Autodesk Inventor part; units mm, degrees
(part 3 of 4)
sketch "Sketch4" plane through (0, 2, 0) normal (0, 1, 0) x (1, 0, 0)
  line L0 (-144.19, 379.14) -> (-144.19, 0) projected
  line L1 (0, 379.14) -> (-144.19, 379.14) projected
  line L2 (-131.665, 24.5025) -> (-131.665, 37.5025)
  line L3 (-117.665, 24.5025) -> (-117.665, 37.5025)
  line L4 (-131.165, 24.0025) -> (-118.165, 24.0025)
  line L5 (-131.165, 38.0025) -> (-118.165, 38.0025)
  arc A0 (-131.665, 24.5025) -> (-131.165, 24.0025) centre (-131.165, 24.5025) ccw
  arc A1 (-131.165, 38.0025) -> (-131.665, 37.5025) centre (-131.165, 37.5025) ccw
  arc A2 (-118.165, 24.0025) -> (-117.665, 24.5025) centre (-118.165, 24.5025) ccw
  arc A3 (-117.665, 37.5025) -> (-118.165, 38.0025) centre (-118.165, 37.5025) ccw
  line L6 (-131.665, 62.6025) -> (-131.665, 75.6025)
  line L7 (-117.665, 62.6025) -> (-117.665, 75.6025)
  line L8 (-131.165, 62.1025) -> (-118.165, 62.1025)
  line L9 (-131.165, 76.1025) -> (-118.165, 76.1025)
  arc A4 (-131.665, 62.6025) -> (-131.165, 62.1025) centre (-131.165, 62.6025) ccw
  arc A5 (-131.165, 76.1025) -> (-131.665, 75.6025) centre (-131.165, 75.6025) ccw
  arc A6 (-118.165, 62.1025) -> (-117.665, 62.6025) centre (-118.165, 62.6025) ccw
  arc A7 (-117.665, 75.6025) -> (-118.165, 76.1025) centre (-118.165, 75.6025) ccw
  line L10 (-131.665, 81.6525) -> (-131.665, 94.6525)
  line L11 (-117.665, 81.6525) -> (-117.665, 94.6525)
  line L12 (-131.165, 81.1525) -> (-118.165, 81.1525)
  line L13 (-131.165, 95.1525) -> (-118.165, 95.1525)
  arc A8 (-131.665, 81.6525) -> (-131.165, 81.1525) centre (-131.165, 81.6525) ccw
  arc A9 (-131.165, 95.1525) -> (-131.665, 94.6525) centre (-131.165, 94.6525) ccw
  arc A10 (-118.165, 81.1525) -> (-117.665, 81.6525) centre (-118.165, 81.6525) ccw
  arc A11 (-117.665, 94.6525) -> (-118.165, 95.1525) centre (-118.165, 94.6525) ccw
  line L14 (-131.665, 100.7025) -> (-131.665, 113.7025)
  line L15 (-117.665, 100.7025) -> (-117.665, 113.7025)
  line L16 (-131.165, 100.2025) -> (-118.165, 100.2025)
  line L17 (-131.165, 114.2025) -> (-118.165, 114.2025)
  arc A12 (-131.665, 100.7025) -> (-131.165, 100.2025) centre (-131.165, 100.7025) ccw
  arc A13 (-131.165, 114.2025) -> (-131.665, 113.7025) centre (-131.165, 113.7025) ccw
  arc A14 (-118.165, 100.2025) -> (-117.665, 100.7025) centre (-118.165, 100.7025) ccw
  arc A15 (-117.665, 113.7025) -> (-118.165, 114.2025) centre (-118.165, 113.7025) ccw
  line L18 (-131.665, 119.7525) -> (-131.665, 132.7525)
  line L19 (-117.665, 119.7525) -> (-117.665, 132.7525)
  line L20 (-131.165, 119.2525) -> (-118.165, 119.2525)
  line L21 (-131.165, 133.2525) -> (-118.165, 133.2525)
  arc A16 (-131.665, 119.7525) -> (-131.165, 119.2525) centre (-131.165, 119.7525) ccw
  arc A17 (-131.165, 133.2525) -> (-131.665, 132.7525) centre (-131.165, 132.7525) ccw
  arc A18 (-118.165, 119.2525) -> (-117.665, 119.7525) centre (-118.165, 119.7525) ccw
  arc A19 (-117.665, 132.7525) -> (-118.165, 133.2525) centre (-118.165, 132.7525) ccw
  line L22 (-131.665, 148.3275) -> (-131.665, 161.3275)
  line L23 (-117.665, 148.3275) -> (-117.665, 161.3275)
  line L24 (-131.165, 147.8275) -> (-118.165, 147.8275)
  line L25 (-131.165, 161.8275) -> (-118.165, 161.8275)
  arc A20 (-131.665, 148.3275) -> (-131.165, 147.8275) centre (-131.165, 148.3275) ccw
  arc A21 (-131.165, 161.8275) -> (-131.665, 161.3275) centre (-131.165, 161.3275) ccw
  arc A22 (-118.165, 147.8275) -> (-117.665, 148.3275) centre (-118.165, 148.3275) ccw
  arc A23 (-117.665, 161.3275) -> (-118.165, 161.8275) centre (-118.165, 161.3275) ccw
  line L26 (-131.665, 167.3775) -> (-131.665, 180.3775)
  line L27 (-117.665, 167.3775) -> (-117.665, 180.3775)
  line L28 (-131.165, 166.8775) -> (-118.165, 166.8775)
  line L29 (-131.165, 180.8775) -> (-118.165, 180.8775)
  arc A24 (-131.665, 167.3775) -> (-131.165, 166.8775) centre (-131.165, 167.3775) ccw
  arc A25 (-131.165, 180.8775) -> (-131.665, 180.3775) centre (-131.165, 180.3775) ccw
  arc A26 (-118.165, 166.8775) -> (-117.665, 167.3775) centre (-118.165, 167.3775) ccw
  arc A27 (-117.665, 180.3775) -> (-118.165, 180.8775) centre (-118.165, 180.3775) ccw
  line L30 (-131.665, 186.4275) -> (-131.665, 199.4275)
  line L31 (-117.665, 186.4275) -> (-117.665, 199.4275)
  line L32 (-131.165, 185.9275) -> (-118.165, 185.9275)
  line L33 (-131.165, 199.9275) -> (-118.165, 199.9275)
  arc A28 (-131.665, 186.4275) -> (-131.165, 185.9275) centre (-131.165, 186.4275) ccw
  arc A29 (-131.165, 199.9275) -> (-131.665, 199.4275) centre (-131.165, 199.4275) ccw
  arc A30 (-118.165, 185.9275) -> (-117.665, 186.4275) centre (-118.165, 186.4275) ccw
  arc A31 (-117.665, 199.4275) -> (-118.165, 199.9275) centre (-118.165, 199.4275) ccw
  line L34 (-131.665, 205.4775) -> (-131.665, 218.4775)
  line L35 (-117.665, 205.4775) -> (-117.665, 218.4775)
  line L36 (-131.165, 204.9775) -> (-118.165, 204.9775)
  line L37 (-131.165, 218.9775) -> (-118.165, 218.9775)
  arc A32 (-131.665, 205.4775) -> (-131.165, 204.9775) centre (-131.165, 205.4775) ccw
  arc A33 (-131.165, 218.9775) -> (-131.665, 218.4775) centre (-131.165, 218.4775) ccw
  arc A34 (-118.165, 204.9775) -> (-117.665, 205.4775) centre (-118.165, 205.4775) ccw
  arc A35 (-117.665, 218.4775) -> (-118.165, 218.9775) centre (-118.165, 218.4775) ccw
  line L38 (-131.665, 234.0525) -> (-131.665, 247.0525)
  line L39 (-117.665, 234.0525) -> (-117.665, 247.0525)
  line L40 (-131.165, 233.5525) -> (-118.165, 233.5525)
  line L41 (-131.165, 247.5525) -> (-118.165, 247.5525)
  arc A36 (-131.665, 234.0525) -> (-131.165, 233.5525) centre (-131.165, 234.0525) ccw
  arc A37 (-131.165, 247.5525) -> (-131.665, 247.0525) centre (-131.165, 247.0525) ccw
  arc A38 (-118.165, 233.5525) -> (-117.665, 234.0525) centre (-118.165, 234.0525) ccw
  arc A39 (-117.665, 247.0525) -> (-118.165, 247.5525) centre (-118.165, 247.0525) ccw
  line L42 (-131.665, 253.1025) -> (-131.665, 266.1025)
  line L43 (-117.665, 253.1025) -> (-117.665, 266.1025)
  line L44 (-131.165, 252.6025) -> (-118.165, 252.6025)
  line L45 (-131.165, 266.6025) -> (-118.165, 266.6025)
  arc A40 (-131.665, 253.1025) -> (-131.165, 252.6025) centre (-131.165, 253.1025) ccw
  arc A41 (-131.165, 266.6025) -> (-131.665, 266.1025) centre (-131.165, 266.1025) ccw
  arc A42 (-118.165, 252.6025) -> (-117.665, 253.1025) centre (-118.165, 253.1025) ccw
  arc A43 (-117.665, 266.1025) -> (-118.165, 266.6025) centre (-118.165, 266.1025) ccw
  line L46 (-131.665, 272.1525) -> (-131.665, 285.1525)
  line L47 (-117.665, 272.1525) -> (-117.665, 285.1525)
  line L48 (-131.165, 271.6525) -> (-118.165, 271.6525)
  line L49 (-131.165, 285.6525) -> (-118.165, 285.6525)
  arc A44 (-131.665, 272.1525) -> (-131.165, 271.6525) centre (-131.165, 272.1525) ccw
  arc A45 (-131.165, 285.6525) -> (-131.665, 285.1525) centre (-131.165, 285.1525) ccw
  arc A46 (-118.165, 271.6525) -> (-117.665, 272.1525) centre (-118.165, 272.1525) ccw
  arc A47 (-117.665, 285.1525) -> (-118.165, 285.6525) centre (-118.165, 285.1525) ccw
  line L50 (-131.665, 291.2025) -> (-131.665, 304.2025)
  line L51 (-117.665, 291.2025) -> (-117.665, 304.2025)
  line L52 (-131.165, 290.7025) -> (-118.165, 290.7025)
  line L53 (-131.165, 304.7025) -> (-118.165, 304.7025)
  arc A48 (-131.665, 291.2025) -> (-131.165, 290.7025) centre (-131.165, 291.2025) ccw
  arc A49 (-131.165, 304.7025) -> (-131.665, 304.2025) centre (-131.165, 304.2025) ccw
  arc A50 (-118.165, 290.7025) -> (-117.665, 291.2025) centre (-118.165, 291.2025) ccw
  arc A51 (-117.665, 304.2025) -> (-118.165, 304.7025) centre (-118.165, 304.2025) ccw
  line L54 (-107.8525, 24.5025) -> (-107.8525, 37.5025)
  line L55 (-93.8525, 24.5025) -> (-93.8525, 37.5025)
  line L56 (-107.3525, 24.0025) -> (-94.3525, 24.0025)
  line L57 (-107.3525, 38.0025) -> (-94.3525, 38.0025)
  arc A52 (-107.8525, 24.5025) -> (-107.3525, 24.0025) centre (-107.3525, 24.5025) ccw
  arc A53 (-107.3525, 38.0025) -> (-107.8525, 37.5025) centre (-107.3525, 37.5025) ccw
  arc A54 (-94.3525, 24.0025) -> (-93.8525, 24.5025) centre (-94.3525, 24.5025) ccw
  arc A55 (-93.8525, 37.5025) -> (-94.3525, 38.0025) centre (-94.3525, 37.5025) ccw
  line L58 (-107.8525, 43.5525) -> (-107.8525, 56.5525)
  line L59 (-93.8525, 43.5525) -> (-93.8525, 56.5525)
  line L60 (-107.3525, 43.0525) -> (-94.3525, 43.0525)
  line L61 (-107.3525, 57.0525) -> (-94.3525, 57.0525)
  arc A56 (-107.8525, 43.5525) -> (-107.3525, 43.0525) centre (-107.3525, 43.5525) ccw
  arc A57 (-107.3525, 57.0525) -> (-107.8525, 56.5525) centre (-107.3525, 56.5525) ccw
  arc A58 (-94.3525, 43.0525) -> (-93.8525, 43.5525) centre (-94.3525, 43.5525) ccw
  arc A59 (-93.8525, 56.5525) -> (-94.3525, 57.0525) centre (-94.3525, 56.5525) ccw
  line L62 (-107.8525, 62.6025) -> (-107.8525, 75.6025)
  line L63 (-93.8525, 62.6025) -> (-93.8525, 75.6025)
  line L64 (-107.3525, 62.1025) -> (-94.3525, 62.1025)
  line L65 (-107.3525, 76.1025) -> (-94.3525, 76.1025)
  arc A60 (-107.8525, 62.6025) -> (-107.3525, 62.1025) centre (-107.3525, 62.6025) ccw
  arc A61 (-107.3525, 76.1025) -> (-107.8525, 75.6025) centre (-107.3525, 75.6025) ccw
  arc A62 (-94.3525, 62.1025) -> (-93.8525, 62.6025) centre (-94.3525, 62.6025) ccw
  arc A63 (-93.8525, 75.6025) -> (-94.3525, 76.1025) centre (-94.3525, 75.6025) ccw
  line L66 (-107.8525, 81.6525) -> (-107.8525, 94.6525)
  line L67 (-93.8525, 81.6525) -> (-93.8525, 94.6525)
  line L68 (-107.3525, 81.1525) -> (-94.3525, 81.1525)
  line L69 (-107.3525, 95.1525) -> (-94.3525, 95.1525)
  arc A64 (-107.8525, 81.6525) -> (-107.3525, 81.1525) centre (-107.3525, 81.6525) ccw
  arc A65 (-107.3525, 95.1525) -> (-107.8525, 94.6525) centre (-107.3525, 94.6525) ccw
  arc A66 (-94.3525, 81.1525) -> (-93.8525, 81.6525) centre (-94.3525, 81.6525) ccw
  arc A67 (-93.8525, 94.6525) -> (-94.3525, 95.1525) centre (-94.3525, 94.6525) ccw
  line L70 (-107.8525, 100.7025) -> (-107.8525, 113.7025)
  line L71 (-93.8525, 100.7025) -> (-93.8525, 113.7025)
  line L72 (-107.3525, 100.2025) -> (-94.3525, 100.2025)
  line L73 (-107.3525, 114.2025) -> (-94.3525, 114.2025)
  arc A68 (-107.8525, 100.7025) -> (-107.3525, 100.2025) centre (-107.3525, 100.7025) ccw
  arc A69 (-107.3525, 114.2025) -> (-107.8525, 113.7025) centre (-107.3525, 113.7025) ccw
  arc A70 (-94.3525, 100.2025) -> (-93.8525, 100.7025) centre (-94.3525, 100.7025) ccw
  arc A71 (-93.8525, 113.7025) -> (-94.3525, 114.2025) centre (-94.3525, 113.7025) ccw
  line L74 (-107.8525, 119.7525) -> (-107.8525, 132.7525)
  line L75 (-93.8525, 119.7525) -> (-93.8525, 132.7525)
  line L76 (-107.3525, 119.2525) -> (-94.3525, 119.2525)
  line L77 (-107.3525, 133.2525) -> (-94.3525, 133.2525)
  arc A72 (-107.8525, 119.7525) -> (-107.3525, 119.2525) centre (-107.3525, 119.7525) ccw
  arc A73 (-107.3525, 133.2525) -> (-107.8525, 132.7525) centre (-107.3525, 132.7525) ccw
  arc A74 (-94.3525, 119.2525) -> (-93.8525, 119.7525) centre (-94.3525, 119.7525) ccw
  arc A75 (-93.8525, 132.7525) -> (-94.3525, 133.2525) centre (-94.3525, 132.7525) ccw
  line L78 (-107.8525, 138.8025) -> (-107.8525, 151.8025)
  line L79 (-93.8525, 138.8025) -> (-93.8525, 151.8025)
  line L80 (-107.3525, 138.3025) -> (-94.3525, 138.3025)
  line L81 (-107.3525, 152.3025) -> (-94.3525, 152.3025)
  arc A76 (-107.8525, 138.8025) -> (-107.3525, 138.3025) centre (-107.3525, 138.8025) ccw
  arc A77 (-107.3525, 152.3025) -> (-107.8525, 151.8025) centre (-107.3525, 151.8025) ccw
  arc A78 (-94.3525, 138.3025) -> (-93.8525, 138.8025) centre (-94.3525, 138.8025) ccw
  arc A79 (-93.8525, 151.8025) -> (-94.3525, 152.3025) centre (-94.3525, 151.8025) ccw
  line L82 (-107.8525, 157.8525) -> (-107.8525, 170.8525)
  line L83 (-93.8525, 157.8525) -> (-93.8525, 170.8525)
  line L84 (-107.3525, 157.3525) -> (-94.3525, 157.3525)
  line L85 (-107.3525, 171.3525) -> (-94.3525, 171.3525)
  arc A80 (-107.8525, 157.8525) -> (-107.3525, 157.3525) centre (-107.3525, 157.8525) ccw
  arc A81 (-107.3525, 171.3525) -> (-107.8525, 170.8525) centre (-107.3525, 170.8525) ccw
  arc A82 (-94.3525, 157.3525) -> (-93.8525, 157.8525) centre (-94.3525, 157.8525) ccw
  arc A83 (-93.8525, 170.8525) -> (-94.3525, 171.3525) centre (-94.3525, 170.8525) ccw
  line L86 (-107.8525, 176.9025) -> (-107.8525, 189.9025)
  line L87 (-93.8525, 176.9025) -> (-93.8525, 189.9025)
  line L88 (-107.3525, 176.4025) -> (-94.3525, 176.4025)
  line L89 (-107.3525, 190.4025) -> (-94.3525, 190.4025)
  arc A84 (-107.8525, 176.9025) -> (-107.3525, 176.4025) centre (-107.3525, 176.9025) ccw
  arc A85 (-107.3525, 190.4025) -> (-107.8525, 189.9025) centre (-107.3525, 189.9025) ccw
  arc A86 (-94.3525, 176.4025) -> (-93.8525, 176.9025) centre (-94.3525, 176.9025) ccw
  arc A87 (-93.8525, 189.9025) -> (-94.3525, 190.4025) centre (-94.3525, 189.9025) ccw
  line L90 (-107.8525, 195.9525) -> (-107.8525, 208.9525)
  line L91 (-93.8525, 195.9525) -> (-93.8525, 208.9525)
  line L92 (-107.3525, 195.4525) -> (-94.3525, 195.4525)
  line L93 (-107.3525, 209.4525) -> (-94.3525, 209.4525)
  arc A88 (-107.8525, 195.9525) -> (-107.3525, 195.4525) centre (-107.3525, 195.9525) ccw
  arc A89 (-107.3525, 209.4525) -> (-107.8525, 208.9525) centre (-107.3525, 208.9525) ccw
  arc A90 (-94.3525, 195.4525) -> (-93.8525, 195.9525) centre (-94.3525, 195.9525) ccw
  arc A91 (-93.8525, 208.9525) -> (-94.3525, 209.4525) centre (-94.3525, 208.9525) ccw
  line L94 (-107.8525, 215.0025) -> (-107.8525, 228.0025)
  line L95 (-93.8525, 215.0025) -> (-93.8525, 228.0025)
  line L96 (-107.3525, 214.5025) -> (-94.3525, 214.5025)
  line L97 (-107.3525, 228.5025) -> (-94.3525, 228.5025)
  arc A92 (-107.8525, 215.0025) -> (-107.3525, 214.5025) centre (-107.3525, 215.0025) ccw
  arc A93 (-107.3525, 228.5025) -> (-107.8525, 228.0025) centre (-107.3525, 228.0025) ccw
  arc A94 (-94.3525, 214.5025) -> (-93.8525, 215.0025) centre (-94.3525, 215.0025) ccw
  arc A95 (-93.8525, 228.0025) -> (-94.3525, 228.5025) centre (-94.3525, 228.0025) ccw
  line L98 (-107.8525, 234.0525) -> (-107.8525, 247.0525)
  line L99 (-93.8525, 234.0525) -> (-93.8525, 247.0525)
  line L100 (-107.3525, 233.5525) -> (-94.3525, 233.5525)
  line L101 (-107.3525, 247.5525) -> (-94.3525, 247.5525)
  arc A96 (-107.8525, 234.0525) -> (-107.3525, 233.5525) centre (-107.3525, 234.0525) ccw
  arc A97 (-107.3525, 247.5525) -> (-107.8525, 247.0525) centre (-107.3525, 247.0525) ccw
  arc A98 (-94.3525, 233.5525) -> (-93.8525, 234.0525) centre (-94.3525, 234.0525) ccw
  arc A99 (-93.8525, 247.0525) -> (-94.3525, 247.5525) centre (-94.3525, 247.0525) ccw
  line L102 (-107.8525, 253.1025) -> (-107.8525, 266.1025)
  line L103 (-93.8525, 253.1025) -> (-93.8525, 266.1025)
  line L104 (-107.3525, 252.6025) -> (-94.3525, 252.6025)
  line L105 (-107.3525, 266.6025) -> (-94.3525, 266.6025)
  arc A100 (-107.8525, 253.1025) -> (-107.3525, 252.6025) centre (-107.3525, 253.1025) ccw
  arc A101 (-107.3525, 266.6025) -> (-107.8525, 266.1025) centre (-107.3525, 266.1025) ccw
  arc A102 (-94.3525, 252.6025) -> (-93.8525, 253.1025) centre (-94.3525, 253.1025) ccw
  arc A103 (-93.8525, 266.1025) -> (-94.3525, 266.6025) centre (-94.3525, 266.1025) ccw
  line L106 (-107.8525, 281.6775) -> (-107.8525, 294.6775)
  line L107 (-93.8525, 281.6775) -> (-93.8525, 294.6775)
  line L108 (-107.3525, 281.1775) -> (-94.3525, 281.1775)
  line L109 (-107.3525, 295.1775) -> (-94.3525, 295.1775)
  arc A104 (-107.8525, 281.6775) -> (-107.3525, 281.1775) centre (-107.3525, 281.6775) ccw
  arc A105 (-107.3525, 295.1775) -> (-107.8525, 294.6775) centre (-107.3525, 294.6775) ccw
  arc A106 (-94.3525, 281.1775) -> (-93.8525, 281.6775) centre (-94.3525, 281.6775) ccw
  arc A107 (-93.8525, 294.6775) -> (-94.3525, 295.1775) centre (-94.3525, 294.6775) ccw
  line L110 (-106.8525, 273.2395) -> (-106.8525, 279.2395)
  line L111 (-91.8525, 273.2395) -> (-91.8525, 279.2395)
  line L112 (-106.3525, 272.7395) -> (-92.3525, 272.7395)
  line L113 (-106.3525, 279.7395) -> (-92.3525, 279.7395)
  arc A108 (-106.8525, 273.2395) -> (-106.3525, 272.7395) centre (-106.3525, 273.2395) ccw
  arc A109 (-106.3525, 279.7395) -> (-106.8525, 279.2395) centre (-106.3525, 279.2395) ccw
  arc A110 (-92.3525, 272.7395) -> (-91.8525, 273.2395) centre (-92.3525, 273.2395) ccw
  arc A111 (-91.8525, 279.2395) -> (-92.3525, 279.7395) centre (-92.3525, 279.2395) ccw
  line L114 (-106.8525, 297.1155) -> (-106.8525, 303.1155)
  line L115 (-91.8525, 297.1155) -> (-91.8525, 303.1155)
  line L116 (-106.3525, 296.6155) -> (-92.3525, 296.6155)
  line L117 (-106.3525, 303.6155) -> (-92.3525, 303.6155)
  arc A112 (-106.8525, 297.1155) -> (-106.3525, 296.6155) centre (-106.3525, 297.1155) ccw
  arc A113 (-106.3525, 303.6155) -> (-106.8525, 303.1155) centre (-106.3525, 303.1155) ccw
  arc A114 (-92.3525, 296.6155) -> (-91.8525, 297.1155) centre (-92.3525, 297.1155) ccw
  arc A115 (-91.8525, 303.1155) -> (-92.3525, 303.6155) centre (-92.3525, 303.1155) ccw
  line L118 (-107.8525, 315.015) -> (-107.8525, 328.015)
  line L119 (-93.8525, 315.015) -> (-93.8525, 328.015)
  line L120 (-107.3525, 314.515) -> (-94.3525, 314.515)
  line L121 (-107.3525, 328.515) -> (-94.3525, 328.515)
  arc A116 (-107.8525, 315.015) -> (-107.3525, 314.515) centre (-107.3525, 315.015) ccw
  arc A117 (-107.3525, 328.515) -> (-107.8525, 328.015) centre (-107.3525, 328.015) ccw
  arc A118 (-94.3525, 314.515) -> (-93.8525, 315.015) centre (-94.3525, 315.015) ccw
  arc A119 (-93.8525, 328.015) -> (-94.3525, 328.515) centre (-94.3525, 328.015) ccw
  line L122 (-107.8525, 334.065) -> (-107.8525, 347.065)
  line L123 (-93.8525, 334.065) -> (-93.8525, 347.065)
  line L124 (-107.3525, 333.565) -> (-94.3525, 333.565)
  line L125 (-107.3525, 347.565) -> (-94.3525, 347.565)
  arc A120 (-107.8525, 334.065) -> (-107.3525, 333.565) centre (-107.3525, 334.065) ccw
  arc A121 (-107.3525, 347.565) -> (-107.8525, 347.065) centre (-107.3525, 347.065) ccw
  arc A122 (-94.3525, 333.565) -> (-93.8525, 334.065) centre (-94.3525, 334.065) ccw
  arc A123 (-93.8525, 347.065) -> (-94.3525, 347.565) centre (-94.3525, 347.065) ccw
  line L126 (-107.8525, 353.115) -> (-107.8525, 366.115)
  line L127 (-93.8525, 353.115) -> (-93.8525, 366.115)
  line L128 (-107.3525, 352.615) -> (-94.3525, 352.615)
  line L129 (-107.3525, 366.615) -> (-94.3525, 366.615)
  arc A124 (-107.8525, 353.115) -> (-107.3525, 352.615) centre (-107.3525, 353.115) ccw
  arc A125 (-107.3525, 366.615) -> (-107.8525, 366.115) centre (-107.3525, 366.115) ccw
  arc A126 (-94.3525, 352.615) -> (-93.8525, 353.115) centre (-94.3525, 353.115) ccw
  arc A127 (-93.8525, 366.115) -> (-94.3525, 366.615) centre (-94.3525, 366.115) ccw
  line L130 (-88.8025, 29.265) -> (-88.8025, 42.265)
  line L131 (-74.8025, 29.265) -> (-74.8025, 42.265)
  line L132 (-88.3025, 28.765) -> (-75.3025, 28.765)
  line L133 (-88.3025, 42.765) -> (-75.3025, 42.765)
  arc A128 (-88.8025, 29.265) -> (-88.3025, 28.765) centre (-88.3025, 29.265) ccw
  arc A129 (-88.3025, 42.765) -> (-88.8025, 42.265) centre (-88.3025, 42.265) ccw
  arc A130 (-75.3025, 28.765) -> (-74.8025, 29.265) centre (-75.3025, 29.265) ccw
  arc A131 (-74.8025, 42.265) -> (-75.3025, 42.765) centre (-75.3025, 42.265) ccw
  line L134 (-88.8025, 53.0775) -> (-88.8025, 66.0775)
  line L135 (-74.8025, 53.0775) -> (-74.8025, 66.0775)
  line L136 (-88.3025, 52.5775) -> (-75.3025, 52.5775)
  line L137 (-88.3025, 66.5775) -> (-75.3025, 66.5775)
  arc A132 (-88.8025, 53.0775) -> (-88.3025, 52.5775) centre (-88.3025, 53.0775) ccw
  arc A133 (-88.3025, 66.5775) -> (-88.8025, 66.0775) centre (-88.3025, 66.0775) ccw
  arc A134 (-75.3025, 52.5775) -> (-74.8025, 53.0775) centre (-75.3025, 53.0775) ccw
  arc A135 (-74.8025, 66.0775) -> (-75.3025, 66.5775) centre (-75.3025, 66.0775) ccw
  line L138 (-88.8025, 72.1275) -> (-88.8025, 85.1275)
  line L139 (-74.8025, 72.1275) -> (-74.8025, 85.1275)
  line L140 (-88.3025, 71.6275) -> (-75.3025, 71.6275)
  line L141 (-88.3025, 85.6275) -> (-75.3025, 85.6275)
  arc A136 (-88.8025, 72.1275) -> (-88.3025, 71.6275) centre (-88.3025, 72.1275) ccw
  arc A137 (-88.3025, 85.6275) -> (-88.8025, 85.1275) centre (-88.3025, 85.1275) ccw
  arc A138 (-75.3025, 71.6275) -> (-74.8025, 72.1275) centre (-75.3025, 72.1275) ccw
  arc A139 (-74.8025, 85.1275) -> (-75.3025, 85.6275) centre (-75.3025, 85.1275) ccw
  line L142 (-88.8025, 91.1775) -> (-88.8025, 104.1775)
  line L143 (-74.8025, 91.1775) -> (-74.8025, 104.1775)
  line L144 (-88.3025, 90.6775) -> (-75.3025, 90.6775)
  line L145 (-88.3025, 104.6775) -> (-75.3025, 104.6775)
  arc A140 (-88.8025, 91.1775) -> (-88.3025, 90.6775) centre (-88.3025, 91.1775) ccw
  arc A141 (-88.3025, 104.6775) -> (-88.8025, 104.1775) centre (-88.3025, 104.1775) ccw
  arc A142 (-75.3025, 90.6775) -> (-74.8025, 91.1775) centre (-75.3025, 91.1775) ccw
  arc A143 (-74.8025, 104.1775) -> (-75.3025, 104.6775) centre (-75.3025, 104.1775) ccw
  line L146 (-88.8025, 110.2275) -> (-88.8025, 123.2275)
  line L147 (-74.8025, 110.2275) -> (-74.8025, 123.2275)
  line L148 (-88.3025, 109.7275) -> (-75.3025, 109.7275)
  line L149 (-88.3025, 123.7275) -> (-75.3025, 123.7275)
  arc A144 (-88.8025, 110.2275) -> (-88.3025, 109.7275) centre (-88.3025, 110.2275) ccw
  arc A145 (-88.3025, 123.7275) -> (-88.8025, 123.2275) centre (-88.3025, 123.2275) ccw
  arc A146 (-75.3025, 109.7275) -> (-74.8025, 110.2275) centre (-75.3025, 110.2275) ccw
  arc A147 (-74.8025, 123.2275) -> (-75.3025, 123.7275) centre (-75.3025, 123.2275) ccw
  line L150 (-88.8025, 129.2775) -> (-88.8025, 142.2775)
  line L151 (-74.8025, 129.2775) -> (-74.8025, 142.2775)
  line L152 (-88.3025, 128.7775) -> (-75.3025, 128.7775)
  line L153 (-88.3025, 142.7775) -> (-75.3025, 142.7775)
  arc A148 (-88.8025, 129.2775) -> (-88.3025, 128.7775) centre (-88.3025, 129.2775) ccw
  arc A149 (-88.3025, 142.7775) -> (-88.8025, 142.2775) centre (-88.3025, 142.2775) ccw
  arc A150 (-75.3025, 128.7775) -> (-74.8025, 129.2775) centre (-75.3025, 129.2775) ccw
  arc A151 (-74.8025, 142.2775) -> (-75.3025, 142.7775) centre (-75.3025, 142.2775) ccw
  line L154 (-88.8025, 148.3275) -> (-88.8025, 161.3275)
  line L155 (-74.8025, 148.3275) -> (-74.8025, 161.3275)
  line L156 (-88.3025, 147.8275) -> (-75.3025, 147.8275)
  line L157 (-88.3025, 161.8275) -> (-75.3025, 161.8275)
  arc A152 (-88.8025, 148.3275) -> (-88.3025, 147.8275) centre (-88.3025, 148.3275) ccw
  arc A153 (-88.3025, 161.8275) -> (-88.8025, 161.3275) centre (-88.3025, 161.3275) ccw
  arc A154 (-75.3025, 147.8275) -> (-74.8025, 148.3275) centre (-75.3025, 148.3275) ccw
  arc A155 (-74.8025, 161.3275) -> (-75.3025, 161.8275) centre (-75.3025, 161.3275) ccw
  line L158 (-88.8025, 167.3775) -> (-88.8025, 180.3775)
  line L159 (-74.8025, 167.3775) -> (-74.8025, 180.3775)
  line L160 (-88.3025, 166.8775) -> (-75.3025, 166.8775)
  line L161 (-88.3025, 180.8775) -> (-75.3025, 180.8775)
  arc A156 (-88.8025, 167.3775) -> (-88.3025, 166.8775) centre (-88.3025, 167.3775) ccw
  arc A157 (-88.3025, 180.8775) -> (-88.8025, 180.3775) centre (-88.3025, 180.3775) ccw
  arc A158 (-75.3025, 166.8775) -> (-74.8025, 167.3775) centre (-75.3025, 167.3775) ccw
  arc A159 (-74.8025, 180.3775) -> (-75.3025, 180.8775) centre (-75.3025, 180.3775) ccw
  line L162 (-88.8025, 186.4275) -> (-88.8025, 199.4275)
  line L163 (-74.8025, 186.4275) -> (-74.8025, 199.4275)
  line L164 (-88.3025, 185.9275) -> (-75.3025, 185.9275)
  line L165 (-88.3025, 199.9275) -> (-75.3025, 199.9275)
  arc A160 (-88.8025, 186.4275) -> (-88.3025, 185.9275) centre (-88.3025, 186.4275) ccw
  arc A161 (-88.3025, 199.9275) -> (-88.8025, 199.4275) centre (-88.3025, 199.4275) ccw
  arc A162 (-75.3025, 185.9275) -> (-74.8025, 186.4275) centre (-75.3025, 186.4275) ccw
  arc A163 (-74.8025, 199.4275) -> (-75.3025, 199.9275) centre (-75.3025, 199.4275) ccw
  line L166 (-88.8025, 205.4775) -> (-88.8025, 218.4775)
  line L167 (-74.8025, 205.4775) -> (-74.8025, 218.4775)
  line L168 (-88.3025, 204.9775) -> (-75.3025, 204.9775)
  line L169 (-88.3025, 218.9775) -> (-75.3025, 218.9775)
  arc A164 (-88.8025, 205.4775) -> (-88.3025, 204.9775) centre (-88.3025, 205.4775) ccw
  arc A165 (-88.3025, 218.9775) -> (-88.8025, 218.4775) centre (-88.3025, 218.4775) ccw
  arc A166 (-75.3025, 204.9775) -> (-74.8025, 205.4775) centre (-75.3025, 205.4775) ccw
  arc A167 (-74.8025, 218.4775) -> (-75.3025, 218.9775) centre (-75.3025, 218.4775) ccw
  line L170 (-88.8025, 224.5275) -> (-88.8025, 237.5275)
  line L171 (-74.8025, 224.5275) -> (-74.8025, 237.5275)
  line L172 (-88.3025, 224.0275) -> (-75.3025, 224.0275)
  line L173 (-88.3025, 238.0275) -> (-75.3025, 238.0275)
  arc A168 (-88.8025, 224.5275) -> (-88.3025, 224.0275) centre (-88.3025, 224.5275) ccw
  arc A169 (-88.3025, 238.0275) -> (-88.8025, 237.5275) centre (-88.3025, 237.5275) ccw
  arc A170 (-75.3025, 224.0275) -> (-74.8025, 224.5275) centre (-75.3025, 224.5275) ccw
  arc A171 (-74.8025, 237.5275) -> (-75.3025, 238.0275) centre (-75.3025, 237.5275) ccw
  line L174 (-88.8025, 243.5775) -> (-88.8025, 256.5775)
  line L175 (-74.8025, 243.5775) -> (-74.8025, 256.5775)
  line L176 (-88.3025, 243.0775) -> (-75.3025, 243.0775)
  line L177 (-88.3025, 257.0775) -> (-75.3025, 257.0775)
  arc A172 (-88.8025, 243.5775) -> (-88.3025, 243.0775) centre (-88.3025, 243.5775) ccw
  arc A173 (-88.3025, 257.0775) -> (-88.8025, 256.5775) centre (-88.3025, 256.5775) ccw
  arc A174 (-75.3025, 243.0775) -> (-74.8025, 243.5775) centre (-75.3025, 243.5775) ccw
  arc A175 (-74.8025, 256.5775) -> (-75.3025, 257.0775) centre (-75.3025, 256.5775) ccw
  line L178 (-88.8025, 262.6275) -> (-88.8025, 275.6275)
  line L179 (-74.8025, 262.6275) -> (-74.8025, 275.6275)
  line L180 (-88.3025, 262.1275) -> (-75.3025, 262.1275)
  line L181 (-88.3025, 276.1275) -> (-75.3025, 276.1275)
  arc A176 (-88.8025, 262.6275) -> (-88.3025, 262.1275) centre (-88.3025, 262.6275) ccw
  arc A177 (-88.3025, 276.1275) -> (-88.8025, 275.6275) centre (-88.3025, 275.6275) ccw
  arc A178 (-75.3025, 262.1275) -> (-74.8025, 262.6275) centre (-75.3025, 262.6275) ccw
  arc A179 (-74.8025, 275.6275) -> (-75.3025, 276.1275) centre (-75.3025, 275.6275) ccw
  line L182 (-88.8025, 286.44) -> (-88.8025, 299.44)
  line L183 (-74.8025, 286.44) -> (-74.8025, 299.44)
  line L184 (-88.3025, 285.94) -> (-75.3025, 285.94)
  line L185 (-88.3025, 299.94) -> (-75.3025, 299.94)
  arc A180 (-88.8025, 286.44) -> (-88.3025, 285.94) centre (-88.3025, 286.44) ccw
  arc A181 (-88.3025, 299.94) -> (-88.8025, 299.44) centre (-88.3025, 299.44) ccw
  arc A182 (-75.3025, 285.94) -> (-74.8025, 286.44) centre (-75.3025, 286.44) ccw
  arc A183 (-74.8025, 299.44) -> (-75.3025, 299.94) centre (-75.3025, 299.44) ccw
  line L186 (-88.8025, 315.015) -> (-88.8025, 328.015)
  line L187 (-74.8025, 315.015) -> (-74.8025, 328.015)
  line L188 (-88.3025, 314.515) -> (-75.3025, 314.515)
  line L189 (-88.3025, 328.515) -> (-75.3025, 328.515)
  arc A184 (-88.8025, 315.015) -> (-88.3025, 314.515) centre (-88.3025, 315.015) ccw
  arc A185 (-88.3025, 328.515) -> (-88.8025, 328.015) centre (-88.3025, 328.015) ccw
  arc A186 (-75.3025, 314.515) -> (-74.8025, 315.015) centre (-75.3025, 315.015) ccw
  arc A187 (-74.8025, 328.015) -> (-75.3025, 328.515) centre (-75.3025, 328.015) ccw
  line L190 (-88.8025, 334.065) -> (-88.8025, 347.065)
  line L191 (-74.8025, 334.065) -> (-74.8025, 347.065)
  line L192 (-88.3025, 333.565) -> (-75.3025, 333.565)
  line L193 (-88.3025, 347.565) -> (-75.3025, 347.565)
  arc A188 (-88.8025, 334.065) -> (-88.3025, 333.565) centre (-88.3025, 334.065) ccw
  arc A189 (-88.3025, 347.565) -> (-88.8025, 347.065) centre (-88.3025, 347.065) ccw
  arc A190 (-75.3025, 333.565) -> (-74.8025, 334.065) centre (-75.3025, 334.065) ccw
  arc A191 (-74.8025, 347.065) -> (-75.3025, 347.565) centre (-75.3025, 347.065) ccw
  line L194 (-88.8025, 353.115) -> (-88.8025, 366.115)
  line L195 (-74.8025, 353.115) -> (-74.8025, 366.115)
  line L196 (-88.3025, 352.615) -> (-75.3025, 352.615)
  line L197 (-88.3025, 366.615) -> (-75.3025, 366.615)
  arc A192 (-88.8025, 353.115) -> (-88.3025, 352.615) centre (-88.3025, 353.115) ccw
  arc A193 (-88.3025, 366.615) -> (-88.8025, 366.115) centre (-88.3025, 366.115) ccw
  arc A194 (-75.3025, 352.615) -> (-74.8025, 353.115) centre (-75.3025, 353.115) ccw
  arc A195 (-74.8025, 366.115) -> (-75.3025, 366.615) centre (-75.3025, 366.115) ccw
  line L198 (-69.7525, 31.6462) -> (-69.7525, 44.6462)
  line L199 (-55.7525, 31.6462) -> (-55.7525, 44.6462)
  line L200 (-69.2525, 31.1462) -> (-56.2525, 31.1462)
  line L201 (-69.2525, 45.1462) -> (-56.2525, 45.1462)
  arc A196 (-69.7525, 31.6462) -> (-69.2525, 31.1462) centre (-69.2525, 31.6462) ccw
  arc A197 (-69.2525, 45.1462) -> (-69.7525, 44.6462) centre (-69.2525, 44.6462) ccw
  arc A198 (-56.2525, 31.1462) -> (-55.7525, 31.6462) centre (-56.2525, 31.6462) ccw
  arc A199 (-55.7525, 44.6462) -> (-56.2525, 45.1462) centre (-56.2525, 44.6462) ccw
  line L202 (-69.7525, 57.84) -> (-69.7525, 70.84)
  line L203 (-55.7525, 57.84) -> (-55.7525, 70.84)
  line L204 (-69.2525, 57.34) -> (-56.2525, 57.34)
  line L205 (-69.2525, 71.34) -> (-56.2525, 71.34)
  arc A200 (-69.7525, 57.84) -> (-69.2525, 57.34) centre (-69.2525, 57.84) ccw
  arc A201 (-69.2525, 71.34) -> (-69.7525, 70.84) centre (-69.2525, 70.84) ccw
  arc A202 (-56.2525, 57.34) -> (-55.7525, 57.84) centre (-56.2525, 57.84) ccw
  arc A203 (-55.7525, 70.84) -> (-56.2525, 71.34) centre (-56.2525, 70.84) ccw
  line L206 (-69.7525, 76.89) -> (-69.7525, 89.89)
  line L207 (-55.7525, 76.89) -> (-55.7525, 89.89)
  line L208 (-69.2525, 76.39) -> (-56.2525, 76.39)
  line L209 (-69.2525, 90.39) -> (-56.2525, 90.39)
  arc A204 (-69.7525, 76.89) -> (-69.2525, 76.39) centre (-69.2525, 76.89) ccw
  arc A205 (-69.2525, 90.39) -> (-69.7525, 89.89) centre (-69.2525, 89.89) ccw
  arc A206 (-56.2525, 76.39) -> (-55.7525, 76.89) centre (-56.2525, 76.89) ccw
  arc A207 (-55.7525, 89.89) -> (-56.2525, 90.39) centre (-56.2525, 89.89) ccw
  line L210 (-69.7525, 95.94) -> (-69.7525, 108.94)
  line L211 (-55.7525, 95.94) -> (-55.7525, 108.94)
  line L212 (-69.2525, 95.44) -> (-56.2525, 95.44)
  line L213 (-69.2525, 109.44) -> (-56.2525, 109.44)
  arc A208 (-69.7525, 95.94) -> (-69.2525, 95.44) centre (-69.2525, 95.94) ccw
  arc A209 (-69.2525, 109.44) -> (-69.7525, 108.94) centre (-69.2525, 108.94) ccw
  arc A210 (-56.2525, 95.44) -> (-55.7525, 95.94) centre (-56.2525, 95.94) ccw
  arc A211 (-55.7525, 108.94) -> (-56.2525, 109.44) centre (-56.2525, 108.94) ccw
  line L214 (-69.7525, 114.99) -> (-69.7525, 127.99)
  line L215 (-55.7525, 114.99) -> (-55.7525, 127.99)
  line L216 (-69.2525, 114.49) -> (-56.2525, 114.49)
  line L217 (-69.2525, 128.49) -> (-56.2525, 128.49)
  arc A212 (-69.7525, 114.99) -> (-69.2525, 114.49) centre (-69.2525, 114.99) ccw
  arc A213 (-69.2525, 128.49) -> (-69.7525, 127.99) centre (-69.2525, 127.99) ccw
  arc A214 (-56.2525, 114.49) -> (-55.7525, 114.99) centre (-56.2525, 114.99) ccw
  arc A215 (-55.7525, 127.99) -> (-56.2525, 128.49) centre (-56.2525, 127.99) ccw
  line L218 (-69.7525, 134.04) -> (-69.7525, 147.04)
  line L219 (-55.7525, 134.04) -> (-55.7525, 147.04)
  line L220 (-69.2525, 133.54) -> (-56.2525, 133.54)
  line L221 (-69.2525, 147.54) -> (-56.2525, 147.54)
  arc A216 (-69.7525, 134.04) -> (-69.2525, 133.54) centre (-69.2525, 134.04) ccw
  arc A217 (-69.2525, 147.54) -> (-69.7525, 147.04) centre (-69.2525, 147.04) ccw
  arc A218 (-56.2525, 133.54) -> (-55.7525, 134.04) centre (-56.2525, 134.04) ccw
  arc A219 (-55.7525, 147.04) -> (-56.2525, 147.54) centre (-56.2525, 147.04) ccw
  line L222 (-69.7525, 153.09) -> (-69.7525, 166.09)
  line L223 (-55.7525, 153.09) -> (-55.7525, 166.09)
  line L224 (-69.2525, 152.59) -> (-56.2525, 152.59)
  line L225 (-69.2525, 166.59) -> (-56.2525, 166.59)
  arc A220 (-69.7525, 153.09) -> (-69.2525, 152.59) centre (-69.2525, 153.09) ccw
  arc A221 (-69.2525, 166.59) -> (-69.7525, 166.09) centre (-69.2525, 166.09) ccw
  arc A222 (-56.2525, 152.59) -> (-55.7525, 153.09) centre (-56.2525, 153.09) ccw
  arc A223 (-55.7525, 166.09) -> (-56.2525, 166.59) centre (-56.2525, 166.09) ccw
  line L226 (-69.7525, 172.14) -> (-69.7525, 185.14)
  line L227 (-55.7525, 172.14) -> (-55.7525, 185.14)
  line L228 (-69.2525, 171.64) -> (-56.2525, 171.64)
  line L229 (-69.2525, 185.64) -> (-56.2525, 185.64)
  arc A224 (-69.7525, 172.14) -> (-69.2525, 171.64) centre (-69.2525, 172.14) ccw
  arc A225 (-69.2525, 185.64) -> (-69.7525, 185.14) centre (-69.2525, 185.14) ccw
  arc A226 (-56.2525, 171.64) -> (-55.7525, 172.14) centre (-56.2525, 172.14) ccw
  arc A227 (-55.7525, 185.14) -> (-56.2525, 185.64) centre (-56.2525, 185.14) ccw
  line L230 (-69.7525, 191.19) -> (-69.7525, 204.19)
  line L231 (-55.7525, 191.19) -> (-55.7525, 204.19)
  line L232 (-69.2525, 190.69) -> (-56.2525, 190.69)
  line L233 (-69.2525, 204.69) -> (-56.2525, 204.69)
  arc A228 (-69.7525, 191.19) -> (-69.2525, 190.69) centre (-69.2525, 191.19) ccw
  arc A229 (-69.2525, 204.69) -> (-69.7525, 204.19) centre (-69.2525, 204.19) ccw
  arc A230 (-56.2525, 190.69) -> (-55.7525, 191.19) centre (-56.2525, 191.19) ccw
  arc A231 (-55.7525, 204.19) -> (-56.2525, 204.69) centre (-56.2525, 204.19) ccw
  line L234 (-69.7525, 210.24) -> (-69.7525, 223.24)
  line L235 (-55.7525, 210.24) -> (-55.7525, 223.24)
  line L236 (-69.2525, 209.74) -> (-56.2525, 209.74)
  line L237 (-69.2525, 223.74) -> (-56.2525, 223.74)
  arc A232 (-69.7525, 210.24) -> (-69.2525, 209.74) centre (-69.2525, 210.24) ccw
  arc A233 (-69.2525, 223.74) -> (-69.7525, 223.24) centre (-69.2525, 223.24) ccw
  arc A234 (-56.2525, 209.74) -> (-55.7525, 210.24) centre (-56.2525, 210.24) ccw
  arc A235 (-55.7525, 223.24) -> (-56.2525, 223.74) centre (-56.2525, 223.24) ccw
  line L238 (-69.7525, 229.29) -> (-69.7525, 242.29)
  line L239 (-55.7525, 229.29) -> (-55.7525, 242.29)
  line L240 (-69.2525, 228.79) -> (-56.2525, 228.79)
  line L241 (-69.2525, 242.79) -> (-56.2525, 242.79)
  arc A236 (-69.7525, 229.29) -> (-69.2525, 228.79) centre (-69.2525, 229.29) ccw
  arc A237 (-69.2525, 242.79) -> (-69.7525, 242.29) centre (-69.2525, 242.29) ccw
  arc A238 (-56.2525, 228.79) -> (-55.7525, 229.29) centre (-56.2525, 229.29) ccw
  arc A239 (-55.7525, 242.29) -> (-56.2525, 242.79) centre (-56.2525, 242.29) ccw
  line L242 (-69.7525, 248.34) -> (-69.7525, 261.34)
  line L243 (-55.7525, 248.34) -> (-55.7525, 261.34)
  line L244 (-69.2525, 247.84) -> (-56.2525, 247.84)
  line L245 (-69.2525, 261.84) -> (-56.2525, 261.84)
  arc A240 (-69.7525, 248.34) -> (-69.2525, 247.84) centre (-69.2525, 248.34) ccw
  arc A241 (-69.2525, 261.84) -> (-69.7525, 261.34) centre (-69.2525, 261.34) ccw
  arc A242 (-56.2525, 247.84) -> (-55.7525, 248.34) centre (-56.2525, 248.34) ccw
  arc A243 (-55.7525, 261.34) -> (-56.2525, 261.84) centre (-56.2525, 261.34) ccw
  line L246 (-69.7525, 279.2962) -> (-69.7525, 292.2962)
  line L247 (-55.7525, 279.2962) -> (-55.7525, 292.2962)
  line L248 (-69.2525, 278.7962) -> (-56.2525, 278.7962)
  line L249 (-69.2525, 292.7962) -> (-56.2525, 292.7962)
  arc A244 (-69.7525, 279.2962) -> (-69.2525, 278.7962) centre (-69.2525, 279.2962) ccw
  arc A245 (-69.2525, 292.7962) -> (-69.7525, 292.2962) centre (-69.2525, 292.2962) ccw
  arc A246 (-56.2525, 278.7962) -> (-55.7525, 279.2962) centre (-56.2525, 279.2962) ccw
  arc A247 (-55.7525, 292.2962) -> (-56.2525, 292.7962) centre (-56.2525, 292.2962) ccw
  line L250 (-68.7525, 270.8582) -> (-68.7525, 276.8582)
  line L251 (-53.7525, 270.8582) -> (-53.7525, 276.8582)
  line L252 (-68.2525, 270.3582) -> (-54.2525, 270.3582)
  line L253 (-68.2525, 277.3582) -> (-54.2525, 277.3582)
  arc A248 (-68.7525, 270.8582) -> (-68.2525, 270.3582) centre (-68.2525, 270.8582) ccw
  arc A249 (-68.2525, 277.3582) -> (-68.7525, 276.8582) centre (-68.2525, 276.8582) ccw
  arc A250 (-54.2525, 270.3582) -> (-53.7525, 270.8582) centre (-54.2525, 270.8582) ccw
  arc A251 (-53.7525, 276.8582) -> (-54.2525, 277.3582) centre (-54.2525, 276.8582) ccw
  line L254 (-68.7525, 294.7342) -> (-68.7525, 300.7342)
  line L255 (-53.7525, 294.7342) -> (-53.7525, 300.7342)
  line L256 (-68.2525, 294.2342) -> (-54.2525, 294.2342)
  line L257 (-68.2525, 301.2342) -> (-54.2525, 301.2342)
  arc A252 (-68.7525, 294.7342) -> (-68.2525, 294.2342) centre (-68.2525, 294.7342) ccw
  arc A253 (-68.2525, 301.2342) -> (-68.7525, 300.7342) centre (-68.2525, 300.7342) ccw
  arc A254 (-54.2525, 294.2342) -> (-53.7525, 294.7342) centre (-54.2525, 294.7342) ccw
  arc A255 (-53.7525, 300.7342) -> (-54.2525, 301.2342) centre (-54.2525, 300.7342) ccw
  line L258 (-50.7025, 36.4087) -> (-50.7025, 49.4087)
  line L259 (-36.7025, 36.4087) -> (-36.7025, 49.4087)
  line L260 (-50.2025, 35.9087) -> (-37.2025, 35.9087)
  line L261 (-50.2025, 49.9087) -> (-37.2025, 49.9087)
  arc A256 (-50.7025, 36.4087) -> (-50.2025, 35.9087) centre (-50.2025, 36.4087) ccw
  arc A257 (-50.2025, 49.9087) -> (-50.7025, 49.4087) centre (-50.2025, 49.4087) ccw
  arc A258 (-37.2025, 35.9087) -> (-36.7025, 36.4087) centre (-37.2025, 36.4087) ccw
  arc A259 (-36.7025, 49.4087) -> (-37.2025, 49.9087) centre (-37.2025, 49.4087) ccw
  line L262 (-49.7025, 27.9707) -> (-49.7025, 33.9707)
  line L263 (-34.7025, 27.9707) -> (-34.7025, 33.9707)
  line L264 (-49.2025, 27.4707) -> (-35.2025, 27.4707)
  line L265 (-49.2025, 34.4707) -> (-35.2025, 34.4707)
  arc A260 (-49.7025, 27.9707) -> (-49.2025, 27.4707) centre (-49.2025, 27.9707) ccw
  arc A261 (-49.2025, 34.4707) -> (-49.7025, 33.9707) centre (-49.2025, 33.9707) ccw
  arc A262 (-35.2025, 27.4707) -> (-34.7025, 27.9707) centre (-35.2025, 27.9707) ccw
  arc A263 (-34.7025, 33.9707) -> (-35.2025, 34.4707) centre (-35.2025, 33.9707) ccw
  line L266 (-49.7025, 51.8467) -> (-49.7025, 57.8467)
  line L267 (-34.7025, 51.8467) -> (-34.7025, 57.8467)
  line L268 (-49.2025, 51.3467) -> (-35.2025, 51.3467)
  line L269 (-49.2025, 58.3467) -> (-35.2025, 58.3467)
  arc A264 (-49.7025, 51.8467) -> (-49.2025, 51.3467) centre (-49.2025, 51.8467) ccw
  arc A265 (-49.2025, 58.3467) -> (-49.7025, 57.8467) centre (-49.2025, 57.8467) ccw
  arc A266 (-35.2025, 51.3467) -> (-34.7025, 51.8467) centre (-35.2025, 51.8467) ccw
  arc A267 (-34.7025, 57.8467) -> (-35.2025, 58.3467) centre (-35.2025, 57.8467) ccw
  line L270 (-50.7025, 67.365) -> (-50.7025, 80.365)
  line L271 (-36.7025, 67.365) -> (-36.7025, 80.365)
  line L272 (-50.2025, 66.865) -> (-37.2025, 66.865)
  line L273 (-50.2025, 80.865) -> (-37.2025, 80.865)
  arc A268 (-50.7025, 67.365) -> (-50.2025, 66.865) centre (-50.2025, 67.365) ccw
  arc A269 (-50.2025, 80.865) -> (-50.7025, 80.365) centre (-50.2025, 80.365) ccw
  arc A270 (-37.2025, 66.865) -> (-36.7025, 67.365) centre (-37.2025, 67.365) ccw
  arc A271 (-36.7025, 80.365) -> (-37.2025, 80.865) centre (-37.2025, 80.365) ccw
  line L274 (-50.7025, 86.415) -> (-50.7025, 99.415)
  line L275 (-36.7025, 86.415) -> (-36.7025, 99.415)
  line L276 (-50.2025, 85.915) -> (-37.2025, 85.915)
  line L277 (-50.2025, 99.915) -> (-37.2025, 99.915)
  arc A272 (-50.7025, 86.415) -> (-50.2025, 85.915) centre (-50.2025, 86.415) ccw
  arc A273 (-50.2025, 99.915) -> (-50.7025, 99.415) centre (-50.2025, 99.415) ccw
  arc A274 (-37.2025, 85.915) -> (-36.7025, 86.415) centre (-37.2025, 86.415) ccw
  arc A275 (-36.7025, 99.415) -> (-37.2025, 99.915) centre (-37.2025, 99.415) ccw
  line L278 (-50.7025, 105.465) -> (-50.7025, 118.465)
  line L279 (-36.7025, 105.465) -> (-36.7025, 118.465)
  line L280 (-50.2025, 104.965) -> (-37.2025, 104.965)
  line L281 (-50.2025, 118.965) -> (-37.2025, 118.965)
  arc A276 (-50.7025, 105.465) -> (-50.2025, 104.965) centre (-50.2025, 105.465) ccw
  arc A277 (-50.2025, 118.965) -> (-50.7025, 118.465) centre (-50.2025, 118.465) ccw
  arc A278 (-37.2025, 104.965) -> (-36.7025, 105.465) centre (-37.2025, 105.465) ccw
  arc A279 (-36.7025, 118.465) -> (-37.2025, 118.965) centre (-37.2025, 118.465) ccw
  line L282 (-50.7025, 124.515) -> (-50.7025, 137.515)
  line L283 (-36.7025, 124.515) -> (-36.7025, 137.515)
  line L284 (-50.2025, 124.015) -> (-37.2025, 124.015)
  line L285 (-50.2025, 138.015) -> (-37.2025, 138.015)
  arc A280 (-50.7025, 124.515) -> (-50.2025, 124.015) centre (-50.2025, 124.515) ccw
  arc A281 (-50.2025, 138.015) -> (-50.7025, 137.515) centre (-50.2025, 137.515) ccw
  arc A282 (-37.2025, 124.015) -> (-36.7025, 124.515) centre (-37.2025, 124.515) ccw
  arc A283 (-36.7025, 137.515) -> (-37.2025, 138.015) centre (-37.2025, 137.515) ccw
  line L286 (-50.7025, 143.565) -> (-50.7025, 156.565)
  line L287 (-36.7025, 143.565) -> (-36.7025, 156.565)
  line L288 (-50.2025, 143.065) -> (-37.2025, 143.065)
  line L289 (-50.2025, 157.065) -> (-37.2025, 157.065)
  arc A284 (-50.7025, 143.565) -> (-50.2025, 143.065) centre (-50.2025, 143.565) ccw
  arc A285 (-50.2025, 157.065) -> (-50.7025, 156.565) centre (-50.2025, 156.565) ccw
  arc A286 (-37.2025, 143.065) -> (-36.7025, 143.565) centre (-37.2025, 143.565) ccw
  arc A287 (-36.7025, 156.565) -> (-37.2025, 157.065) centre (-37.2025, 156.565) ccw
  line L290 (-50.7025, 162.615) -> (-50.7025, 175.615)
  line L291 (-36.7025, 162.615) -> (-36.7025, 175.615)
  line L292 (-50.2025, 162.115) -> (-37.2025, 162.115)
  line L293 (-50.2025, 176.115) -> (-37.2025, 176.115)
  arc A288 (-50.7025, 162.615) -> (-50.2025, 162.115) centre (-50.2025, 162.615) ccw
  arc A289 (-50.2025, 176.115) -> (-50.7025, 175.615) centre (-50.2025, 175.615) ccw
  arc A290 (-37.2025, 162.115) -> (-36.7025, 162.615) centre (-37.2025, 162.615) ccw
  arc A291 (-36.7025, 175.615) -> (-37.2025, 176.115) centre (-37.2025, 175.615) ccw
  line L294 (-50.7025, 181.665) -> (-50.7025, 194.665)
  line L295 (-36.7025, 181.665) -> (-36.7025, 194.665)
  line L296 (-50.2025, 181.165) -> (-37.2025, 181.165)
  line L297 (-50.2025, 195.165) -> (-37.2025, 195.165)
  arc A292 (-50.7025, 181.665) -> (-50.2025, 181.165) centre (-50.2025, 181.665) ccw
  arc A293 (-50.2025, 195.165) -> (-50.7025, 194.665) centre (-50.2025, 194.665) ccw
  arc A294 (-37.2025, 181.165) -> (-36.7025, 181.665) centre (-37.2025, 181.665) ccw
  arc A295 (-36.7025, 194.665) -> (-37.2025, 195.165) centre (-37.2025, 194.665) ccw
  line L298 (-50.7025, 200.715) -> (-50.7025, 213.715)
  line L299 (-36.7025, 200.715) -> (-36.7025, 213.715)
  line L300 (-50.2025, 200.215) -> (-37.2025, 200.215)
  line L301 (-50.2025, 214.215) -> (-37.2025, 214.215)
  arc A296 (-50.7025, 200.715) -> (-50.2025, 200.215) centre (-50.2025, 200.715) ccw
  arc A297 (-50.2025, 214.215) -> (-50.7025, 213.715) centre (-50.2025, 213.715) ccw
  arc A298 (-37.2025, 200.215) -> (-36.7025, 200.715) centre (-37.2025, 200.715) ccw
  arc A299 (-36.7025, 213.715) -> (-37.2025, 214.215) centre (-37.2025, 213.715) ccw
  line L302 (-50.7025, 219.765) -> (-50.7025, 232.765)
  line L303 (-36.7025, 219.765) -> (-36.7025, 232.765)
  line L304 (-50.2025, 219.265) -> (-37.2025, 219.265)
  line L305 (-50.2025, 233.265) -> (-37.2025, 233.265)
  arc A300 (-50.7025, 219.765) -> (-50.2025, 219.265) centre (-50.2025, 219.765) ccw
  arc A301 (-50.2025, 233.265) -> (-50.7025, 232.765) centre (-50.2025, 232.765) ccw
  arc A302 (-37.2025, 219.265) -> (-36.7025, 219.765) centre (-37.2025, 219.765) ccw
  arc A303 (-36.7025, 232.765) -> (-37.2025, 233.265) centre (-37.2025, 232.765) ccw
  line L306 (-50.7025, 238.815) -> (-50.7025, 251.815)
  line L307 (-36.7025, 238.815) -> (-36.7025, 251.815)
  line L308 (-50.2025, 238.315) -> (-37.2025, 238.315)
  line L309 (-50.2025, 252.315) -> (-37.2025, 252.315)
  arc A304 (-50.7025, 238.815) -> (-50.2025, 238.315) centre (-50.2025, 238.815) ccw
  arc A305 (-50.2025, 252.315) -> (-50.7025, 251.815) centre (-50.2025, 251.815) ccw
  arc A306 (-37.2025, 238.315) -> (-36.7025, 238.815) centre (-37.2025, 238.815) ccw
  arc A307 (-36.7025, 251.815) -> (-37.2025, 252.315) centre (-37.2025, 251.815) ccw
  line L310 (-50.7025, 274.5337) -> (-50.7025, 287.5337)
  line L311 (-36.7025, 274.5337) -> (-36.7025, 287.5337)
  line L312 (-50.2025, 274.0337) -> (-37.2025, 274.0337)
  line L313 (-50.2025, 288.0337) -> (-37.2025, 288.0337)
  arc A308 (-50.7025, 274.5337) -> (-50.2025, 274.0337) centre (-50.2025, 274.5337) ccw
  arc A309 (-50.2025, 288.0337) -> (-50.7025, 287.5337) centre (-50.2025, 287.5337) ccw
  arc A310 (-37.2025, 274.0337) -> (-36.7025, 274.5337) centre (-37.2025, 274.5337) ccw
  arc A311 (-36.7025, 287.5337) -> (-37.2025, 288.0337) centre (-37.2025, 287.5337) ccw
  line L314 (-49.7025, 266.0957) -> (-49.7025, 272.0957)
  line L315 (-34.7025, 266.0957) -> (-34.7025, 272.0957)
  line L316 (-49.2025, 265.5957) -> (-35.2025, 265.5957)
  line L317 (-49.2025, 272.5957) -> (-35.2025, 272.5957)
  arc A312 (-49.7025, 266.0957) -> (-49.2025, 265.5957) centre (-49.2025, 266.0957) ccw
  arc A313 (-49.2025, 272.5957) -> (-49.7025, 272.0957) centre (-49.2025, 272.0957) ccw
  arc A314 (-35.2025, 265.5957) -> (-34.7025, 266.0957) centre (-35.2025, 266.0957) ccw
  arc A315 (-34.7025, 272.0957) -> (-35.2025, 272.5957) centre (-35.2025, 272.0957) ccw
  line L318 (-49.7025, 289.9717) -> (-49.7025, 295.9717)
  line L319 (-34.7025, 289.9717) -> (-34.7025, 295.9718)
  line L320 (-49.2025, 289.4717) -> (-35.2025, 289.4717)
  line L321 (-49.2025, 296.4717) -> (-35.2025, 296.4717)
  arc A316 (-49.7025, 289.9717) -> (-49.2025, 289.4717) centre (-49.2025, 289.9717) ccw
  arc A317 (-49.2025, 296.4717) -> (-49.7025, 295.9717) centre (-49.2025, 295.9717) ccw
  arc A318 (-35.2025, 289.4717) -> (-34.7025, 289.9717) centre (-35.2025, 289.9717) ccw
  arc A319 (-34.7025, 295.9718) -> (-35.2025, 296.4717) centre (-35.2025, 295.9718) ccw
  line L322 (-50.7025, 334.065) -> (-50.7025, 347.065)
  line L323 (-36.7025, 334.065) -> (-36.7025, 347.065)
  line L324 (-50.2025, 333.565) -> (-37.2025, 333.565)
  line L325 (-50.2025, 347.565) -> (-37.2025, 347.565)
  arc A320 (-50.7025, 334.065) -> (-50.2025, 333.565) centre (-50.2025, 334.065) ccw
  arc A321 (-50.2025, 347.565) -> (-50.7025, 347.065) centre (-50.2025, 347.065) ccw
  arc A322 (-37.2025, 333.565) -> (-36.7025, 334.065) centre (-37.2025, 334.065) ccw
  arc A323 (-36.7025, 347.065) -> (-37.2025, 347.565) centre (-37.2025, 347.065) ccw
  line L326 (-31.6525, 26.8837) -> (-31.6525, 39.8837)
  line L327 (-17.6525, 26.8837) -> (-17.6525, 39.8837)
  line L328 (-31.1525, 26.3837) -> (-18.1525, 26.3837)
  line L329 (-31.1525, 40.3837) -> (-18.1525, 40.3837)
  arc A324 (-31.6525, 26.8837) -> (-31.1525, 26.3837) centre (-31.1525, 26.8837) ccw
  arc A325 (-31.1525, 40.3837) -> (-31.6525, 39.8837) centre (-31.1525, 39.8837) ccw
  arc A326 (-18.1525, 26.3837) -> (-17.6525, 26.8837) centre (-18.1525, 26.8837) ccw
  arc A327 (-17.6525, 39.8837) -> (-18.1525, 40.3837) centre (-18.1525, 39.8837) ccw
  line L330 (-31.6525, 50.6962) -> (-31.6525, 63.6962)
  line L331 (-17.6525, 50.6962) -> (-17.6525, 63.6962)
  line L332 (-31.1525, 50.1962) -> (-18.1525, 50.1962)
  line L333 (-31.1525, 64.1962) -> (-18.1525, 64.1962)
  arc A328 (-31.6525, 50.6962) -> (-31.1525, 50.1962) centre (-31.1525, 50.6962) ccw
  arc A329 (-31.1525, 64.1962) -> (-31.6525, 63.6962) centre (-31.1525, 63.6962) ccw
  arc A330 (-18.1525, 50.1962) -> (-17.6525, 50.6962) centre (-18.1525, 50.6962) ccw
  arc A331 (-17.6525, 63.6962) -> (-18.1525, 64.1962) centre (-18.1525, 63.6962) ccw
  line L334 (-31.6525, 74.5087) -> (-31.6525, 87.5087)
  line L335 (-17.6525, 74.5087) -> (-17.6525, 87.5087)
  line L336 (-31.1525, 74.0087) -> (-18.1525, 74.0087)
  line L337 (-31.1525, 88.0087) -> (-18.1525, 88.0087)
  arc A332 (-31.6525, 74.5087) -> (-31.1525, 74.0087) centre (-31.1525, 74.5087) ccw
  arc A333 (-31.1525, 88.0087) -> (-31.6525, 87.5087) centre (-31.1525, 87.5087) ccw
  arc A334 (-18.1525, 74.0087) -> (-17.6525, 74.5087) centre (-18.1525, 74.5087) ccw
  arc A335 (-17.6525, 87.5087) -> (-18.1525, 88.0087) centre (-18.1525, 87.5087) ccw
  line L338 (-31.6525, 145.9462) -> (-31.6525, 158.9462)
  line L339 (-17.6525, 145.9462) -> (-17.6525, 158.9462)
  line L340 (-31.1525, 145.4462) -> (-18.1525, 145.4462)
  line L341 (-31.1525, 159.4462) -> (-18.1525, 159.4462)
  arc A336 (-31.6525, 145.9462) -> (-31.1525, 145.4462) centre (-31.1525, 145.9462) ccw
  arc A337 (-31.1525, 159.4462) -> (-31.6525, 158.9462) centre (-31.1525, 158.9462) ccw
  arc A338 (-18.1525, 145.4462) -> (-17.6525, 145.9462) centre (-18.1525, 145.9462) ccw
  arc A339 (-17.6525, 158.9462) -> (-18.1525, 159.4462) centre (-18.1525, 158.9462) ccw
  line L342 (-30.6525, 99.4462) -> (-30.6525, 105.4462)
  line L343 (-15.6525, 99.4462) -> (-15.6525, 105.4462)
  line L344 (-30.1525, 98.9462) -> (-16.1525, 98.9462)
  line L345 (-30.1525, 105.9462) -> (-16.1525, 105.9462)
  arc A340 (-30.6525, 99.4462) -> (-30.1525, 98.9462) centre (-30.1525, 99.4462) ccw
  arc A341 (-30.1525, 105.9462) -> (-30.6525, 105.4462) centre (-30.1525, 105.4462) ccw
  arc A342 (-16.1525, 98.9462) -> (-15.6525, 99.4462) centre (-16.1525, 99.4462) ccw
  arc A343 (-15.6525, 105.4462) -> (-16.1525, 105.9462) centre (-16.1525, 105.4462) ccw
  line L346 (-30.6525, 199.4462) -> (-30.6525, 205.4462)
  line L347 (-15.6525, 199.4462) -> (-15.6525, 205.4462)
  line L348 (-30.1525, 198.9462) -> (-16.1525, 198.9462)
  line L349 (-30.1525, 205.9462) -> (-16.1525, 205.9462)
  arc A344 (-30.6525, 199.4462) -> (-30.1525, 198.9462) centre (-30.1525, 199.4462) ccw
  arc A345 (-30.1525, 205.9462) -> (-30.6525, 205.4462) centre (-30.1525, 205.4462) ccw
  arc A346 (-16.1525, 198.9462) -> (-15.6525, 199.4462) centre (-16.1525, 199.4462) ccw
  arc A347 (-15.6525, 205.4462) -> (-16.1525, 205.9462) centre (-16.1525, 205.4462) ccw
  line L350 (-31.6525, 217.3837) -> (-31.6525, 230.3837)
  line L351 (-17.6525, 217.3837) -> (-17.6525, 230.3837)
  line L352 (-31.1525, 216.8837) -> (-18.1525, 216.8837)
  line L353 (-31.1525, 230.8837) -> (-18.1525, 230.8837)
  arc A348 (-31.6525, 217.3837) -> (-31.1525, 216.8837) centre (-31.1525, 217.3837) ccw
  arc A349 (-31.1525, 230.8837) -> (-31.6525, 230.3837) centre (-31.1525, 230.3837) ccw
  arc A350 (-18.1525, 216.8837) -> (-17.6525, 217.3837) centre (-18.1525, 217.3837) ccw
  arc A351 (-17.6525, 230.3837) -> (-18.1525, 230.8837) centre (-18.1525, 230.3837) ccw